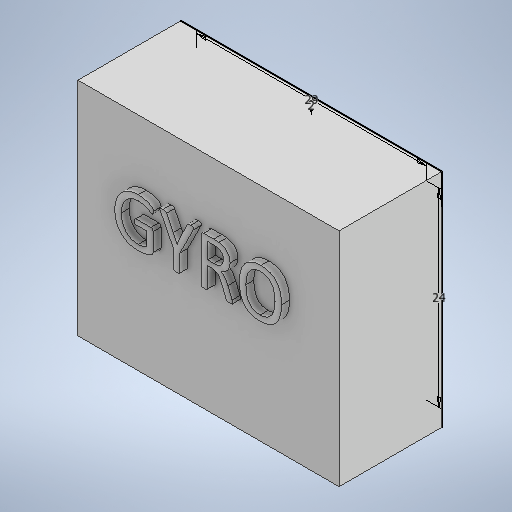
# Autodesk Inventor part: cover
Saved by Autodesk Inventor 2025.2 (Build 292293000, 293)
## iProperties
Created: 2025-03-05
Part Number: cover
Material: Generic
Document SubType Name: Modeling
Designer: cutterj
Density: 1 g/cm^3
Appearance: Default
Author: cutterj
Autodesk Inventor part; units mm, degrees
ref_plane "YZ Plane" through (0, 0, 0) normal (1, 0, 0) x (0, 1, 0)
ref_plane "XZ Plane" through (0, 0, 0) normal (0, 1, 0) x (-1, 0, 0)
ref_plane "XY Plane" through (0, 0, 0) normal (0, 0, 1) x (1, 0, 0)
sketch "Sketch1" plane through (0, 0, 0) normal (0, 0, 1) x (1, 0, 0)
  line L0 (0, 0) -> (29, 0)
  line L1 (29, 0) -> (29, 24)
  line L2 (29, 24) -> (0, 24)
  line L3 (0, 24) -> (0, 0)
  line L4 (-2, 26) -> (31, 26)
  line L5 (31, 26) -> (31, -2)
  line L6 (31, -2) -> (-2, -2)
  line L7 (-2, -2) -> (-2, 26)
  dimension "d0" = 29
  dimension "d1" = 24
  dimension "d2" = 2
  constraints: 16 end point, 4 parallel, 2 perpendicular, 1 horizontal, 3 other
  measures "d0" distance of L2.end L1.end
  measures "d1" distance of L1.end L0.end
  measures "d2" distance between parallel lines of L2 L4
extrude "Extrusion1" add sketch "Sketch1" along normal blind 13 contours L3 L2 L1 L0 | L4 L5 L6 L7
extrude "Extrusion2" cut sketch "Sketch1" along normal blind 11 contours L3 L2 L1 L0
sketch "Sketch2" plane through (0, 0, 13) normal (0, 0, 1) x (1, 0, 0)
  line L0 (3.2257, 18.2769) -> (25.4363, 18.2769) construction
  line L1 (25.4363, 18.2769) -> (25.4363, 7.9924) construction
  line L2 (25.4363, 7.9924) -> (3.2257, 7.9924) construction
  line L3 (3.2257, 7.9924) -> (3.2257, 18.2769) construction
  spline S0 degree 2 poles (8.5046, 17.3811) (8.5046, 17.291) (8.4877, 17.1558) (8.4482, 17.0713) (8.3919, 17.0319) (8.3637, 17.0319) knots 0 0 0 1 2 3 4 4 4
  spline S1 degree 2 poles (8.3637, 17.0319) (8.3074, 17.0319) (8.0482, 17.2065) (7.6144, 17.4206) (7.0116, 17.5952) (6.5947, 17.5952) knots 0 0 0 1 2 3 4 4 4
  spline S2 degree 2 poles (6.5947, 17.5952) (6.0989, 17.5952) (5.3158, 17.2347) (4.775, 16.598) (4.482, 15.7192) (4.482, 15.2065) knots 0 0 0 1 2 3 4 4 4
  spline S3 degree 2 poles (4.482, 15.2065) (4.482, 14.6319) (4.8031, 13.7473) (5.3609, 13.1389) (6.144, 12.8234) (6.6116, 12.8234) knots 0 0 0 1 2 3 4 4 4
  spline S4 degree 2 poles (6.6116, 12.8234) (6.8877, 12.8234) (7.4567, 12.9586) (7.6989, 13.0882) knots 0 0 0 1 2 2 2
  line L4 (7.6989, 13.0882) -> (7.6989, 14.829)
  line L5 (7.6989, 14.829) -> (6.313, 14.829)
  spline S5 degree 2 poles (6.313, 14.829) (6.2341, 14.829) (6.1553, 14.9868) (6.1553, 15.1558) knots 0 0 0 1 2 2 2
  spline S6 degree 2 poles (6.1553, 15.1558) (6.1553, 15.2403) (6.1722, 15.3642) (6.2172, 15.4431) (6.2736, 15.4826) (6.313, 15.4826) knots 0 0 0 1 2 3 4 4 4
  line L6 (6.313, 15.4826) -> (8.2116, 15.4826)
  spline S7 degree 2 poles (8.2116, 15.4826) (8.2623, 15.4826) (8.3637, 15.4431) (8.4482, 15.3699) (8.4933, 15.2403) (8.4933, 15.1614) knots 0 0 0 1 2 3 4 4 4
  line L7 (8.4933, 15.1614) -> (8.4933, 12.8854)
  spline S8 degree 2 poles (8.4933, 12.8854) (8.4933, 12.7614) (8.4088, 12.5868) (8.144, 12.4516) (7.7158, 12.2995) (7.2651, 12.1868) (6.8031, 12.1304) (6.5778, 12.1304) knots 0 0 0 1 2 3 4 5 6 6 6
  spline S9 degree 2 poles (6.5778, 12.1304) (5.8848, 12.1304) (4.7975, 12.5586) (4.0426, 13.353) (3.6482, 14.4628) (3.6482, 15.1445) knots 0 0 0 1 2 3 4 4 4
  spline S10 degree 2 poles (3.6482, 15.1445) (3.6482, 15.8544) (4.0764, 17.0093) (4.8539, 17.8262) (5.9468, 18.2713) (6.6116, 18.2713) knots 0 0 0 1 2 3 4 4 4
  spline S11 degree 2 poles (6.6116, 18.2713) (6.9553, 18.2713) (7.5524, 18.153) (8.02, 17.9896) (8.3412, 17.8037) (8.4595, 17.6854) (8.5046, 17.5276) (8.5046, 17.3811) knots 0 0 0 1 2 3 4 5 6 6 6
  line L8 (11.8905, 14.5361) -> (11.8905, 12.3333)
  spline S12 degree 2 poles (11.8905, 12.3333) (11.8905, 12.2995) (11.851, 12.2431) (11.7609, 12.2093) (11.6031, 12.1868) (11.4961, 12.1868) knots 0 0 0 1 2 3 4 4 4
  spline S13 degree 2 poles (11.4961, 12.1868) (11.3834, 12.1868) (11.2313, 12.2093) (11.1355, 12.2431) (11.0961, 12.2995) (11.0961, 12.3333) knots 0 0 0 1 2 3 4 4 4
  line L9 (11.0961, 12.3333) -> (11.0961, 14.5361)
  line L10 (11.0961, 14.5361) -> (9.406, 17.9051)
  spline S14 degree 2 poles (9.406, 17.9051) (9.3553, 18.0121) (9.3327, 18.1304) (9.4003, 18.198) (9.5806, 18.2149) (9.7327, 18.2149) knots 0 0 0 1 2 3 4 4 4
  spline S15 degree 2 poles (9.7327, 18.2149) (9.8736, 18.2149) (10.0426, 18.198) (10.144, 18.1642) (10.1947, 18.1023) (10.2172, 18.0572) knots 0 0 0 1 2 3 4 4 4
  line L11 (10.2172, 18.0572) -> (11.0454, 16.3389)
  spline S16 degree 2 poles (11.0454, 16.3389) (11.1581, 16.0966) (11.3891, 15.5614) (11.5074, 15.291) knots 0 0 0 1 2 2 2
  line L12 (11.5074, 15.291) -> (11.5186, 15.291)
  spline S17 degree 2 poles (11.5186, 15.291) (11.6257, 15.5502) (11.851, 16.0741) (11.9637, 16.3276) knots 0 0 0 1 2 2 2
  line L13 (11.9637, 16.3276) -> (12.7975, 18.0516)
  spline S18 degree 2 poles (12.7975, 18.0516) (12.8088, 18.1023) (12.8595, 18.1642) (12.9496, 18.198) (13.1017, 18.2149) (13.2257, 18.2149) knots 0 0 0 1 2 3 4 4 4
  spline S19 degree 2 poles (13.2257, 18.2149) (13.3891, 18.2149) (13.5806, 18.1924) (13.6539, 18.1248) (13.6313, 18.0065) (13.5806, 17.9051) knots 0 0 0 1 2 3 4 4 4
  line L14 (13.5806, 17.9051) -> (11.8905, 14.5361)
  spline S20 degree 2 poles (18.5778, 12.3333) (18.5778, 12.2995) (18.5496, 12.2431) (18.4595, 12.2037) (18.2905, 12.1868) (18.1553, 12.1868) knots 0 0 0 1 2 3 4 4 4
  spline S21 degree 2 poles (18.1553, 12.1868) (18.0313, 12.1868) (17.8792, 12.2037) (17.7891, 12.2488) (17.7384, 12.322) (17.7215, 12.3783) knots 0 0 0 1 2 3 4 4 4
  line L15 (17.7215, 12.3783) -> (17.1693, 13.7811)
  spline S22 degree 2 poles (17.1693, 13.7811) (17.0736, 14.0234) (16.8651, 14.4234) (16.5778, 14.7107) (16.1947, 14.8741) (15.9186, 14.8741) knots 0 0 0 1 2 3 4 4 4
  line L16 (15.9186, 14.8741) -> (15.3891, 14.8741)
  line L17 (15.3891, 14.8741) -> (15.3891, 12.3333)
  spline S23 degree 2 poles (15.3891, 12.3333) (15.3891, 12.2995) (15.3496, 12.2431) (15.2595, 12.2093) (15.1074, 12.1868) (14.9947, 12.1868) knots 0 0 0 1 2 3 4 4 4
  spline S24 degree 2 poles (14.9947, 12.1868) (14.8764, 12.1868) (14.7243, 12.2093) (14.6341, 12.2431) (14.5947, 12.2995) (14.5947, 12.3333) knots 0 0 0 1 2 3 4 4 4
  line L18 (14.5947, 12.3333) -> (14.5947, 17.8657)
  spline S25 degree 2 poles (14.5947, 17.8657) (14.5947, 18.0459) (14.7862, 18.1868) (14.8877, 18.1868) knots 0 0 0 1 2 2 2
  line L19 (14.8877, 18.1868) -> (16.1609, 18.1868)
  spline S26 degree 2 poles (16.1609, 18.1868) (16.3862, 18.1868) (16.6848, 18.1642) (16.8031, 18.1473) knots 0 0 0 1 2 2 2
  spline S27 degree 2 poles (16.8031, 18.1473) (17.1524, 18.091) (17.682, 17.8319) (18.0426, 17.4319) (18.2229, 16.9192) (18.2229, 16.6093) knots 0 0 0 1 2 3 4 4 4
  spline S28 degree 2 poles (18.2229, 16.6093) (18.2229, 16.3107) (18.0595, 15.8375) (17.7553, 15.4713) (17.3327, 15.2009) (17.0679, 15.1107) knots 0 0 0 1 2 3 4 4 4
  spline S29 degree 2 poles (17.0679, 15.1107) (17.2144, 15.0431) (17.4567, 14.8459) (17.6651, 14.5699) (17.851, 14.2093) (17.9412, 13.984) knots 0 0 0 1 2 3 4 4 4
  line L20 (17.9412, 13.984) -> (18.4764, 12.6713)
  spline S30 degree 2 poles (18.4764, 12.6713) (18.544, 12.5023) (18.5778, 12.3727) (18.5778, 12.3333) knots 0 0 0 1 2 2 2
  spline S31 degree 2 poles (17.3834, 16.5304) (17.3834, 16.8797) (17.0679, 17.3642) (16.7017, 17.4713) knots 0 0 0 1 2 2 2
  spline S32 degree 2 poles (16.7017, 17.4713) (16.5834, 17.5051) (16.2961, 17.5333) (16.0595, 17.5333) knots 0 0 0 1 2 2 2
  line L21 (16.0595, 17.5333) -> (15.3891, 17.5333)
  line L22 (15.3891, 17.5333) -> (15.3891, 15.5164)
  line L23 (15.3891, 15.5164) -> (16.1665, 15.5164)
  spline S33 degree 2 poles (16.1665, 15.5164) (16.4764, 15.5164) (16.9384, 15.6685) (17.2426, 15.9445) (17.3834, 16.3107) (17.3834, 16.5304) knots 0 0 0 1 2 3 4 4 4
  spline S34 degree 2 poles (24.7299, 15.2685) (24.7299, 14.5473) (24.3862, 13.3811) (23.7102, 12.5642) (22.6848, 12.1248) (22.0031, 12.1248) knots 0 0 0 1 2 3 4 4 4
  spline S35 degree 2 poles (22.0031, 12.1248) (21.3271, 12.1248) (20.3468, 12.5248) (19.7046, 13.291) (19.3891, 14.429) (19.3891, 15.1671) knots 0 0 0 1 2 3 4 4 4
  spline S36 degree 2 poles (19.3891, 15.1671) (19.3891, 15.8769) (19.7327, 17.0319) (20.4144, 17.8375) (21.4398, 18.2769) (22.1215, 18.2769) knots 0 0 0 1 2 3 4 4 4
  spline S37 degree 2 poles (22.1215, 18.2769) (22.7806, 18.2769) (23.7609, 17.8826) (24.4088, 17.1164) (24.7299, 15.9952) (24.7299, 15.2685) knots 0 0 0 1 2 3 4 4 4
  spline S38 degree 2 poles (23.8905, 15.2178) (23.8905, 15.7248) (23.7102, 16.598) (23.2933, 17.2403) (22.5891, 17.6009) (22.0708, 17.6009) knots 0 0 0 1 2 3 4 4 4
  spline S39 degree 2 poles (22.0708, 17.6009) (21.5581, 17.6009) (20.8539, 17.2121) (20.42, 16.5642) (20.2285, 15.7023) (20.2285, 15.2234) knots 0 0 0 1 2 3 4 4 4
  spline S40 degree 2 poles (20.2285, 15.2234) (20.2285, 14.6995) (20.4031, 13.8093) (20.82, 13.1671) (21.513, 12.8121) (22.0426, 12.8121) knots 0 0 0 1 2 3 4 4 4
  spline S41 degree 2 poles (22.0426, 12.8121) (22.5609, 12.8121) (23.2708, 13.2009) (23.7046, 13.86) (23.8905, 14.7333) (23.8905, 15.2178) knots 0 0 0 1 2 3 4 4 4
  point P0 (0, 0)
  constraints: 2 other
extrude "Extrusion3" add sketch "Sketch2" along normal blind 1
body "Solid1"
